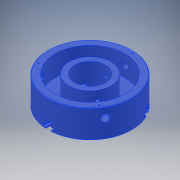
# Autodesk Inventor part: Base
Saved by Autodesk Inventor 2018 (Build 220112000, 112)
## iProperties
Created: 2011-02-15
Part Number: Base
Document SubType Name: Modeling
Designer: nguyenducthang
Density: 1 g/cm^3
Mass: 28.0904 g
Surface Area: 145.179 cm^2
Volume: 28.0904 cm^3
Material: Generic
Appearance: Default
Author: nguyenducthang
Autodesk Inventor part; units mm, degrees
ref_plane "YZ Plane" through (0, 0, 0) normal (1, 0, 0) x (0, 1, 0)
ref_plane "XZ Plane" through (0, 0, 0) normal (0, 1, 0) x (-1, 0, 0)
sketch "Sketch10" plane through (0, 0, 0) normal (0, 0, 1) x (1, 0, 0)
  line L0 (0, 0) -> (0, 23.8782) construction
  line L1 (0, 0) -> (-30, 0)
  line L2 (-30, 0) -> (-30, 20)
  line L3 (-30, 20) -> (-25, 20)
  line L4 (-25, 20) -> (-25, 5)
  line L5 (-25, 5) -> (-15, 5)
  line L6 (-15, 5) -> (-15, 20)
  line L7 (-15, 20) -> (-11, 20)
  line L8 (-11, 20) -> (-11, 0)
  dimension "d51" = 15
  dimension "d52" = 4
  dimension "d53" = 25
  dimension "d54" = 5
  dimension "d55" = 5
  dimension "d56" = 15
  dimension "d69" = 0
  constraints: 18 end point, 4 parallel, 4 perpendicular, 1 point on line, 1 vertical, 1 other
  measures "d51" distance between parallel lines of L6 L0
  measures "d52" distance of L6.end L7.end
  measures "d53" distance between parallel lines of L4 L0
  measures "d54" distance of L2.end L3.end
  measures "d55" distance between parallel lines of L5 L1
  measures "d56" distance between parallel lines of L5 L3
  measures "d69" distance between parallel lines of L3 L7
revolve "Revolution3" add sketch "Sketch10" angle 360 about axis through (0, 0, 0) along (0, 1, 0)
sketch "Sketch11" plane through (0, 0, 0) normal (0, 0, 1) x (1, 0, 0)
  line L0 (30, 20) -> (-30, 20) projected
  line L1 (0, 20) -> (0, -4.7272) construction
  line L2 (-2, 5) -> (-2, 3)
  line L3 (-2, 3) -> (-3.5, 3)
  line L4 (-3.5, 3) -> (-3.5, 1)
  line L5 (-3.5, 1) -> (-2, 1)
  line L6 (-2, 1) -> (-2, 0)
  line L7 (-2, 0) -> (0, 0)
  line L8 (-2, 20) -> (0, 20)
  line L9 (-30, 20) -> (30, 20)
  line L10 (2, 5) -> (2, 3)
  line L11 (2, 3) -> (3.5, 3)
  line L12 (3.5, 3) -> (3.5, 1)
  line L13 (3.5, 1) -> (2, 1)
  line L14 (2, 1) -> (2, 0)
  line L15 (2, 0) -> (0, 0)
  line L16 (2, 20) -> (0, 20)
  line L17 (30, 0) -> (-30, 0) projected
  line L18 (30, 20) -> (-30, 20) projected
  line L19 (30, 0) -> (-30, 0) projected
  line L20 (-2, 5) -> (2, 5)
  line L21 (-2, 5) -> (2, 5) construction
  line L22 (2, 5) -> (2, 6)
  line L23 (2, 6) -> (-2, 6)
  line L24 (-2, 6) -> (-2, 5)
  line L25 (-2, 3) -> (-2, 6)
  line L26 (2, 3) -> (2, 6)
  dimension "d60" = 2
  dimension "d61" = 2
  dimension "d62" = 3.5
  dimension "d63" = 2
  dimension "d64" = 1
  dimension "d67" = 0
  dimension "d68" = 2
  dimension "d86" = 1
  constraints: 46 end point, 8 symmetric about line, 6 parallel, 4 collinear, 4 perpendicular, 3 point on line, 1 horizontal, 1 midpoint
  measures "d60" distance of L6.end L7.end
  measures "d61" distance between parallel lines of L1 L2
  measures "d62" distance between parallel lines of L1 L4
  measures "d63" distance of L3.end L4.end
  measures "d64" distance between parallel lines of L5 L7
  measures "d67" distance between parallel lines of L7 L19
  measures "d68" distance between parallel lines of L20 L3
  measures "d86" distance of L23.end L2.start
extrude "Extrusion8" cut sketch "Sketch11" along normal through all
ref_plane "Work Plane1" through (0, 0, -35) normal (0, 0, 1) x (1, 0, 0)
sketch "Sketch15" plane through (0, 0, 0) normal (0, 0, 1) x (1, 0, 0)
  circle A0 centre (0, 13) radius 1.3292 projected
extrude "Extrusion12" cut sketch "Sketch15" against normal through all
sketch "Sketch16" plane through (0, 20, 0) normal (0, 1, 0) x (1, 0, 0)
  arc A0 (2.5, 28.25) -> (2.5, 27.25) centre (2.5, 27.75) ccw
  circle A1 centre (2.5, 27.75) radius 0.5
  constraints: 2 point on circle, 1 centre point, 1 coincident, 1 vertical alignment, 6 other
extrude "Extrusion13" cut sketch "Sketch16" against normal blind 10
ref_plane "Work Plane2" through (0, 0, -30) normal (0, 0, 1) x (1, 0, 0)
sketch "Sketch17" plane through (0, 0, -30) normal (0, 0, 1) x (1, 0, 0)
  circle A0 centre (0, 13) radius 2.5
  dimension "d83" = 5
  constraints: 1 centre point, 1 coincident
  measures "d83" diameter of A0
extrude "Extrusion14" cut sketch "Sketch17" along normal blind 10
pattern_circular "Circular Pattern1" count 3 over 360 about axis through (0, 10, 0) along (0, 1, 0) of "Extrusion8", "Extrusion12", "Extrusion13", "Extrusion14"
chamfer "Chamfer1" distance 0.4 angle 45 5 edges at (-21.9089, 0, 20.4939) (-29.2206, 0, -6.7938) (25.9808, 0, 15) (0, 0, -30) (30, 20, 0)
body "Solid1"
